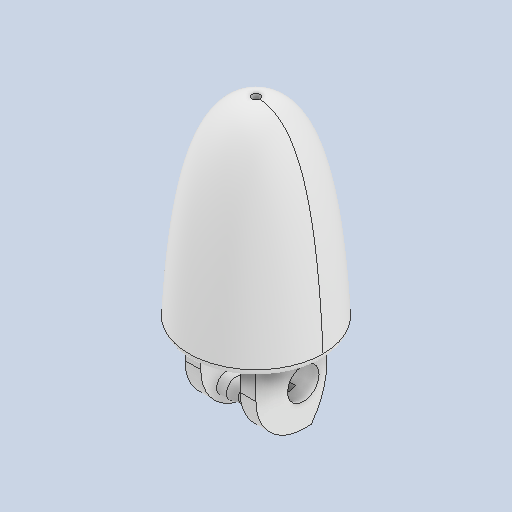
# Autodesk Inventor part: Ring_3
Saved by Autodesk Inventor 2022 (Build 260153000, 153)
## iProperties
Created: 2023-01-15
Part Number: Ring_3
Material: ABS Plastic
Document SubType Name: Modeling
Designer: 48735
Density: 1.06 g/cm^3
Appearance: Smooth - White
Author: 48735
Autodesk Inventor part; units mm, degrees
ref_plane "YZ Plane" through (0, 0, 0) normal (1, 0, 0) x (0, 1, 0)
ref_plane "XZ Plane" through (0, 0, 0) normal (0, 1, 0) x (-1, 0, 0)
sketch "Sketch1" plane through (0, 0, 0) normal (0, 1, 0) x (-1, 0, 0)
  circle A0 centre (0, 0) radius 8.5
  line L0 (0, 0) -> (-2.5, 0)
  line L1 (-2.5, 0) -> (4.5, 0)
  line L2 (4.5, 0) -> (4.5, -2.5)
  line L3 (4.5, -2.5) -> (4.5, 4.5)
  line L4 (-4.5, 0) -> (-4.5, -2.5)
  line L5 (-4.5, 4.5) -> (-4.5, 0)
  line L6 (4.5, -4.5) -> (-4.5, -4.5)
  line L7 (-2.5, -2.5) -> (2.5, -2.5)
  line L8 (-2.5, -2.5) -> (-2.5, 4.5)
  line L9 (-2.5, 4.5) -> (-4.5, 4.5)
  line L10 (2.5, -2.5) -> (2.5, 4.5)
  line L11 (2.5, 4.5) -> (4.5, 4.5)
  line L12 (-4.5, -2.5) -> (-4.5, -4.5)
  line L13 (4.5, -4.5) -> (4.5, -2.5)
  point P0 (6.5, 0)
  constraints: 28 end point, 6 point on line, 5 perpendicular, 3 vertical, 2 horizontal, 1 centre point, 1 coincident, 1 collinear
extrude "Extrusion1" add sketch "Sketch1" along normal blind 10 contours L8 L7 L10 L1 L2 L13 L6 L12 L4 L5 L9 | L10 L11 L3 L1
sketch "Sketch2" plane through (0, 10, 0) normal (0, 1, 0) x (1, 0, 0)
  circle A0 centre (0, 0) radius 8.5
  circle A1 centre (0, 0) radius 1.25
  dimension "d11" = 17
  dimension "d12" = 2.5
  constraints: 2 centre point, 2 coincident
  measures "d11" diameter of A0
  measures "d12" diameter of A1
extrude "Extrusion2" add sketch "Sketch2" along normal blind 1
fillet "Fillet3" radius 1 1 edges at (-8.5, 10, 0)
fillet "Fillet4" radius 1 1 edges at (-1.25, 10, 0)
fillet "Fillet5" radius 6 2 edges at (3.5, 0, 4.5) (-3.5, 0, 4.5)
fillet "Fillet6" radius 10 1 edges at (0, 0, -4.5)
sketch "Sketch3" plane through (-4.5, 10, -4.5) normal (-1, 0, 0) x (0, 0, 1)
  arc A0 (3, -10) -> (9, -4) centre (3, -4) ccw projected
  line L0 (3, -10) -> (3, -5)
  point P0 (4.5, -10)
  dimension "d24" = 5
  constraints: 2 end point, 1 vertical
  measures "d24" distance of L0.start L0.end
hole "Hole1" at (-4.5, 5, -1.5) direction (1, 0, 0) diameter 4 depth 10
sketch "Sketch4" plane through (2.5, 10, -2.5) normal (-1, 0, 0) x (0, 0, 1)
  line L0 (7, -4) -> (7, 0) projected
  circle A0 centre (3.75, -7) radius 1.25
  point P0 (2.5, -10)
  constraints: 1 centre point
extrude "Extrusion3" add sketch "Sketch4" along normal blind 2.5
chamfer "Chamfer1" distance 0.25 distance2 1.25 1 edges at (0, 3, 0) measured on face at (0, 2.3808, 1.5915)
sketch "Sketch5" plane through (-2.5, 10, 4.5) normal (1, 0, 0) x (0, 0, -1)
  circle A0 centre (3.25, -7) radius 1.25 projected
  circle A1 centre (3.25, -7) radius 1.25
  point P0 (4.5, -10)
  constraints: 1 centre point, 1 coincident
extrude "Extrusion4" add sketch "Sketch5" along normal blind 2.5
chamfer "Chamfer2" distance 0.25 distance2 1.25 1 edges at (0, 3, 2.5) measured on face at (0, 2.8205, 0.1051)
ref_plane "Work Plane1" through (-1.25, 11, 0) normal (0, 0, 1) x (1, 0, 0)
sketch "Sketch7" plane through (-1.25, 11, 0) normal (0, 0, 1) x (1, 0, 0)
  line L0 (0, 0) -> (2.5, 0) projected
  line L1 (1.25, 0) -> (1.25, 25)
  line L2 (1.25, 0) -> (1.25, 24)
  line L3 (1.25, 24) -> (6.0871, 24) construction
  line L4 (6.0871, 24) -> (8.9052, 17.9211) construction
  line L5 (9.75, 0) -> (-7.25, 0) projected
  line L6 (8.9052, 17.9211) -> (9.75, 0) construction
  spline S0 degree 3 poles (1.25, 24) (6.0871, 24) (8.9052, 17.9211) (9.75, 0) knots 1 1 1 1 2 2 2 2
  line L7 (9.75, 0) -> (1.25, 0)
  point P0 (1.25, -11)
  dimension "d48" = 25
  dimension "d49" = 24
  constraints: 6 end point, 1 collinear, 1 midpoint, 1 perpendicular, 1 point on line, 1 vertical, 3 other
  measures "d48" distance of L1.start L1.end
  measures "d49" distance of L1.start L2.end
revolve "Revolution1" add sketch "Sketch7" angle 360 about axis through (0, 11, 0) along (0, 1, 0)
sketch "Sketch8" plane through (0, 11, 0) normal (0, -1, 0) x (1, 0, 0)
  circle A0 centre (0, 0) radius 1.25
  constraints: 1 centre point, 1 coincident
hole "Hole2" at (0, 11, 0) direction (0, 1, 0) diameter 1 depth 40
fillet "Fillet7" radius 1 1 edges at (0, 11, 0.5)
body "Solid1"
